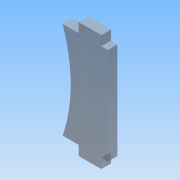
# Autodesk Inventor part: tip_up
Saved by Autodesk Inventor 2015 (Build 190159000, 159)
## iProperties
Created: 2016-01-28
Part Number: tip_up
Material: Plastique PMMA
Document SubType Name: Tôlerie
Designer: Gregwar
Density: 1.188 g/cm^3
Sheet Metal Rule: Par défaut_mm
Appearance: Polycarbonate - Transparent
Author: Gregwar
Autodesk Inventor part; units mm, degrees
ref_plane "YZ Plane" through (0, 0, 0) normal (1, 0, 0) x (0, 1, 0)
ref_plane "XZ Plane" through (0, 0, 0) normal (0, 1, 0) x (-1, 0, 0)
ref_plane "XY Plane" through (0, 0, 0) normal (0, 0, 1) x (1, 0, 0)
sketch "Esquisse1" plane through (0, 0, 0) normal (0, 1, 0) x (-1, 0, 0)
  line L0 (0, 0) -> (14, 0)
  line L1 (14, 0) -> (14, -30)
  line L2 (14, -30) -> (0, -30)
  line L3 (0, -30) -> (0, 0)
  line L4 (2, 0) -> (9, 0)
  line L5 (9, 0) -> (9, 3)
  line L6 (9, 3) -> (2, 3)
  line L7 (2, 3) -> (2, 0)
  line L8 (14, -15) -> (0, -15) construction
  line L9 (2, -30) -> (9, -30)
  line L10 (9, -30) -> (9, -33)
  line L11 (9, -33) -> (2, -33)
  line L12 (2, -33) -> (2, -30)
  dimension "d0" = 2
  dimension "d1" = 3
  dimension "d2" = 30
  dimension "d3" = 7
  dimension "d4" = 5
  measures "d0" distance between parallel lines of L3 L7
  measures "d1" distance of L6.end L4.start
  measures "d2" distance of L2.end L0.start
  measures "d3" distance of L5.end L6.end
  measures "d4" distance between parallel lines of L5 L1
extrude "Plaque1" add sketch "Esquisse1" along normal blind 3
sketch "Esquisse2" plane through (0, 3, 0) normal (0, 1, 0) x (1, 0, 0)
  line L0 (-2, 0) -> (-2, -3) construction
  line L1 (0, 0) -> (-2, 0) construction
  line L2 (0, 30) -> (0, 0) construction
  line L3 (-2, 30) -> (0, 30) construction
  line L4 (-2, 33) -> (-2, 30) construction
  line L5 (-9, 33) -> (-2, 33) construction
  line L6 (-9, 30) -> (-9, 33) construction
  line L7 (-14, 30) -> (-9, 30) construction
  line L8 (-14, 0) -> (-14, 30) construction
  line L9 (-9, 0) -> (-14, 0) construction
  line L10 (-9, -3) -> (-9, 0) construction
  line L11 (-2, -3) -> (-9, -3) construction
  line L12 (-14, 0) -> (-14, 30) construction
  line L13 (-14, 0) -> (-9, 15) construction
  line L14 (-9, 15) -> (-14, 30) construction
  spline S0 degree 2 poles (-14, 0) (-9, 15) (-14, 30) knots 1 1 1 2 2 2
  line L15 (-14, 0) -> (-14, 30)
  line L16 (-9, 15) -> (-14, 15) construction
  line L17 (-14, 0) -> (-14, 30) construction
  dimension "d6" = 5
  constraints: 6 end point, 2 vertical, 1 coincident, 1 midpoint, 1 perpendicular, 3 other
  measures "d6" distance from line of L13.end L8
extrude "Couper1" cut sketch "Esquisse2" against normal blind 3
equation "\"d7\" = Epaisseur"
equation "\"LargeurGrugeage\" = Epaisseur"
equation "\"ProfondeurGrugeage\" = 0.5 * Epaisseur"
equation "\"TailleGrugeage\" = 4 * Epaisseur"
equation "\"RestesMinimum\" = 2 * Epaisseur"
equation "\"Rayondetransition\" = RayonPli"
equation "\"TailleRayonJacobi\" = RayonPli"
equation "\"TailleJeu\" = Epaisseur"
equation "\"d5\" = RayonPli"
equation "\"Epaisseur\" = 3"
equation "\"RayonPli\" = 4"
